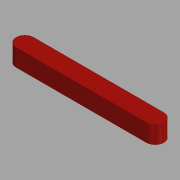
# Autodesk Inventor part: LED red
Saved by Autodesk Inventor 2014 SP2 (Build 180246200, 246)
## iProperties
Created: 2016-01-21
Part Number: LED red
Material: ABS plast
Document SubType Name: Modeling
Designer: Mervart
Mass: 0.0702602 g
Surface Area: 1.3885 cm^2
Volume: 0.0662832 cm^3
Density: 1.06 g/cm^3
Appearance: Oranžovo-červená
LastSaveDate: 21.09.2010
Hmotnost: 0
Author: Mervart
Autodesk Inventor part; units mm, degrees
ref_plane "YZ Plane" through (0, 0, 0) normal (1, 0, 0) x (0, 1, 0)
ref_plane "XZ Plane" through (0, 0, 0) normal (0, 1, 0) x (-1, 0, 0)
ref_plane "XY Plane" through (0, 0, 0) normal (0, 0, 1) x (1, 0, 0)
sketch "Náčrt4" plane through (0, 0, 0) normal (0, 0, 1) x (1, 0, 0)
  line L0 (-32.5599, -1.7649) -> (-17.5599, -1.7649) construction
  line L1 (-17.5599, -3.7649) -> (-32.5599, -3.7649) construction
  line L2 (-50.5599, -1.7649) -> (-35.5599, -1.7649) construction
  line L3 (-35.5599, -3.7649) -> (-50.5599, -3.7649) construction
  line L4 (-68.5599, -1.7649) -> (-53.5599, -1.7649) construction
  line L5 (-53.5599, -3.7649) -> (-68.5599, -3.7649) construction
  line L6 (-68.5599, 11.7351) -> (-9.4199, 11.7351) construction
  arc A0 (-68.5599, 11.7351) -> (-77.8599, 2.4351) centre (-68.5599, 2.4351) ccw construction
  line L7 (-77.8599, -87.5649) -> (-77.8599, 2.4351) construction
  arc A1 (-77.8599, -87.5649) -> (-68.5599, -96.8649) centre (-68.5599, -87.5649) ccw construction
  line L8 (-6.5599, -96.8649) -> (-68.5599, -96.8649) construction
  line L9 (-6.5599, -96.8649) -> (-6.5599, -2.5649) construction
  line L10 (-6.5599, -2.5649) -> (-9.4199, 11.7351) construction
  line L11 (-69.5599, -21.7649) -> (-69.5599, -7.7649) construction
  line L12 (-68.0599, -6.2649) -> (-54.0599, -6.2649) construction
  line L13 (-52.5599, -7.7649) -> (-52.5599, -21.7649) construction
  line L14 (-54.0599, -23.2649) -> (-68.0599, -23.2649) construction
  circle A2 centre (-43.0499, 7.9351) radius 0.3 construction
  circle A3 centre (-39.5499, 4.4351) radius 0.3 construction
  circle A4 centre (-43.0499, 0.9351) radius 0.3 construction
  circle A5 centre (-46.5499, 4.4351) radius 0.3 construction
  circle A6 centre (-43.0499, 4.4351) radius 0.3 construction
  circle A7 centre (-45.5248, 6.9099) radius 0.3 construction
  circle A8 centre (-45.5248, 1.9602) radius 0.3 construction
  circle A9 centre (-40.575, 1.9602) radius 0.3 construction
  circle A10 centre (-40.575, 6.9099) radius 0.3 construction
  line L15 (-32.5599, -1.7649) -> (-17.5599, -1.7649)
  line L16 (-17.5599, -3.7649) -> (-32.5599, -3.7649)
  line L17 (-38.3583, -87.0597) -> (-38.9319, -87.8789) projected
  arc A11 (-38.9319, -87.8789) -> (-47.1879, -87.8789) centre (-43.0599, -93.7743) ccw projected
  line L18 (-47.1879, -87.8789) -> (-47.7615, -87.0597) projected
  arc A12 (-38.3583, -87.0597) -> (-47.7615, -87.0597) centre (-43.0599, -93.7743) ccw projected
  circle A13 centre (-43.0599, -93.7743) radius 0.9 projected
  line L19 (-40.5363, -89.5777) -> (-41.1099, -90.3968) projected
  arc A14 (-41.1099, -90.3968) -> (-45.0099, -90.3968) centre (-43.0599, -93.7743) ccw projected
  line L20 (-45.0099, -90.3968) -> (-45.5835, -89.5777) projected
  arc A15 (-40.5363, -89.5777) -> (-45.5835, -89.5777) centre (-43.0599, -93.7743) ccw projected
  arc A16 (-36.4655, -84.3565) -> (-49.6543, -84.3565) centre (-43.0599, -93.7743) ccw projected
  line L21 (-36.4655, -84.3565) -> (-37.0391, -85.1757) projected
  arc A17 (-37.0391, -85.1757) -> (-49.0807, -85.1757) centre (-43.0599, -93.7743) ccw projected
  line L22 (-49.0807, -85.1757) -> (-49.6543, -84.3565) projected
  line L23 (-33.5599, -75.7649) -> (-33.5599, -61.7649) projected
  arc A18 (-32.0599, -60.2649) -> (-33.5599, -61.7649) centre (-32.0599, -61.7649) ccw projected
  line L24 (-32.0599, -60.2649) -> (-18.0599, -60.2649) projected
  arc A19 (-16.5599, -61.7649) -> (-18.0599, -60.2649) centre (-18.0599, -61.7649) ccw projected
  line L25 (-16.5599, -61.7649) -> (-16.5599, -75.7649) projected
  arc A20 (-18.0599, -77.2649) -> (-16.5599, -75.7649) centre (-18.0599, -75.7649) ccw projected
  line L26 (-18.0599, -77.2649) -> (-32.0599, -77.2649) projected
  arc A21 (-33.5599, -75.7649) -> (-32.0599, -77.2649) centre (-32.0599, -75.7649) ccw projected
  line L27 (-51.5599, -75.7649) -> (-51.5599, -61.7649) projected
  arc A22 (-50.0599, -60.2649) -> (-51.5599, -61.7649) centre (-50.0599, -61.7649) ccw projected
  line L28 (-50.0599, -60.2649) -> (-36.0599, -60.2649) projected
  arc A23 (-34.5599, -61.7649) -> (-36.0599, -60.2649) centre (-36.0599, -61.7649) ccw projected
  line L29 (-34.5599, -61.7649) -> (-34.5599, -75.7649) projected
  arc A24 (-36.0599, -77.2649) -> (-34.5599, -75.7649) centre (-36.0599, -75.7649) ccw projected
  line L30 (-36.0599, -77.2649) -> (-50.0599, -77.2649) projected
  arc A25 (-51.5599, -75.7649) -> (-50.0599, -77.2649) centre (-50.0599, -75.7649) ccw projected
  line L31 (-69.5599, -75.7649) -> (-69.5599, -61.7649) projected
  arc A26 (-68.0599, -60.2649) -> (-69.5599, -61.7649) centre (-68.0599, -61.7649) ccw projected
  line L32 (-68.0599, -60.2649) -> (-54.0599, -60.2649) projected
  arc A27 (-52.5599, -61.7649) -> (-54.0599, -60.2649) centre (-54.0599, -61.7649) ccw projected
  line L33 (-52.5599, -61.7649) -> (-52.5599, -75.7649) projected
  arc A28 (-54.0599, -77.2649) -> (-52.5599, -75.7649) centre (-54.0599, -75.7649) ccw projected
  line L34 (-54.0599, -77.2649) -> (-68.0599, -77.2649) projected
  arc A29 (-69.5599, -75.7649) -> (-68.0599, -77.2649) centre (-68.0599, -75.7649) ccw projected
  line L35 (-33.5599, -57.7649) -> (-33.5599, -43.7649) projected
  arc A30 (-32.0599, -42.2649) -> (-33.5599, -43.7649) centre (-32.0599, -43.7649) ccw projected
  line L36 (-32.0599, -42.2649) -> (-18.0599, -42.2649) projected
  arc A31 (-16.5599, -43.7649) -> (-18.0599, -42.2649) centre (-18.0599, -43.7649) ccw projected
  line L37 (-16.5599, -43.7649) -> (-16.5599, -57.7649) projected
  arc A32 (-18.0599, -59.2649) -> (-16.5599, -57.7649) centre (-18.0599, -57.7649) ccw projected
  line L38 (-18.0599, -59.2649) -> (-32.0599, -59.2649) projected
  arc A33 (-33.5599, -57.7649) -> (-32.0599, -59.2649) centre (-32.0599, -57.7649) ccw projected
  line L39 (-51.5599, -57.7649) -> (-51.5599, -43.7649) projected
  arc A34 (-50.0599, -42.2649) -> (-51.5599, -43.7649) centre (-50.0599, -43.7649) ccw projected
  line L40 (-50.0599, -42.2649) -> (-36.0599, -42.2649) projected
  arc A35 (-34.5599, -43.7649) -> (-36.0599, -42.2649) centre (-36.0599, -43.7649) ccw projected
  line L41 (-34.5599, -43.7649) -> (-34.5599, -57.7649) projected
  arc A36 (-36.0599, -59.2649) -> (-34.5599, -57.7649) centre (-36.0599, -57.7649) ccw projected
  line L42 (-36.0599, -59.2649) -> (-50.0599, -59.2649) projected
  arc A37 (-51.5599, -57.7649) -> (-50.0599, -59.2649) centre (-50.0599, -57.7649) ccw projected
  line L43 (-69.5599, -57.7649) -> (-69.5599, -43.7649) projected
  arc A38 (-68.0599, -42.2649) -> (-69.5599, -43.7649) centre (-68.0599, -43.7649) ccw projected
  line L44 (-68.0599, -42.2649) -> (-54.0599, -42.2649) projected
  arc A39 (-52.5599, -43.7649) -> (-54.0599, -42.2649) centre (-54.0599, -43.7649) ccw projected
  line L45 (-52.5599, -43.7649) -> (-52.5599, -57.7649) projected
  arc A40 (-54.0599, -59.2649) -> (-52.5599, -57.7649) centre (-54.0599, -57.7649) ccw projected
  line L46 (-54.0599, -59.2649) -> (-68.0599, -59.2649) projected
  arc A41 (-69.5599, -57.7649) -> (-68.0599, -59.2649) centre (-68.0599, -57.7649) ccw projected
  line L47 (-33.5599, -39.7649) -> (-33.5599, -25.7649) projected
  arc A42 (-32.0599, -24.2649) -> (-33.5599, -25.7649) centre (-32.0599, -25.7649) ccw projected
  line L48 (-32.0599, -24.2649) -> (-18.0599, -24.2649) projected
  arc A43 (-16.5599, -25.7649) -> (-18.0599, -24.2649) centre (-18.0599, -25.7649) ccw projected
  line L49 (-16.5599, -25.7649) -> (-16.5599, -39.7649) projected
  arc A44 (-18.0599, -41.2649) -> (-16.5599, -39.7649) centre (-18.0599, -39.7649) ccw projected
  line L50 (-18.0599, -41.2649) -> (-32.0599, -41.2649) projected
  arc A45 (-33.5599, -39.7649) -> (-32.0599, -41.2649) centre (-32.0599, -39.7649) ccw projected
  line L51 (-51.5599, -39.7649) -> (-51.5599, -25.7649) projected
  arc A46 (-50.0599, -24.2649) -> (-51.5599, -25.7649) centre (-50.0599, -25.7649) ccw projected
  line L52 (-50.0599, -24.2649) -> (-36.0599, -24.2649) projected
  arc A47 (-34.5599, -25.7649) -> (-36.0599, -24.2649) centre (-36.0599, -25.7649) ccw projected
  line L53 (-34.5599, -25.7649) -> (-34.5599, -39.7649) projected
  arc A48 (-36.0599, -41.2649) -> (-34.5599, -39.7649) centre (-36.0599, -39.7649) ccw projected
  line L54 (-36.0599, -41.2649) -> (-50.0599, -41.2649) projected
  arc A49 (-51.5599, -39.7649) -> (-50.0599, -41.2649) centre (-50.0599, -39.7649) ccw projected
  line L55 (-69.5599, -39.7649) -> (-69.5599, -25.7649) projected
  arc A50 (-68.0599, -24.2649) -> (-69.5599, -25.7649) centre (-68.0599, -25.7649) ccw projected
  line L56 (-68.0599, -24.2649) -> (-54.0599, -24.2649) projected
  arc A51 (-52.5599, -25.7649) -> (-54.0599, -24.2649) centre (-54.0599, -25.7649) ccw projected
  line L57 (-52.5599, -25.7649) -> (-52.5599, -39.7649) projected
  arc A52 (-54.0599, -41.2649) -> (-52.5599, -39.7649) centre (-54.0599, -39.7649) ccw projected
  line L58 (-54.0599, -41.2649) -> (-68.0599, -41.2649) projected
  arc A53 (-69.5599, -39.7649) -> (-68.0599, -41.2649) centre (-68.0599, -39.7649) ccw projected
  line L59 (-33.5599, -21.7649) -> (-33.5599, -7.7649) projected
  arc A54 (-32.0599, -6.2649) -> (-33.5599, -7.7649) centre (-32.0599, -7.7649) ccw projected
  line L60 (-32.0599, -6.2649) -> (-18.0599, -6.2649) projected
  arc A55 (-16.5599, -7.7649) -> (-18.0599, -6.2649) centre (-18.0599, -7.7649) ccw projected
  line L61 (-16.5599, -7.7649) -> (-16.5599, -21.7649) projected
  arc A56 (-18.0599, -23.2649) -> (-16.5599, -21.7649) centre (-18.0599, -21.7649) ccw projected
  line L62 (-18.0599, -23.2649) -> (-32.0599, -23.2649) projected
  arc A57 (-33.5599, -21.7649) -> (-32.0599, -23.2649) centre (-32.0599, -21.7649) ccw projected
  line L63 (-51.5599, -21.7649) -> (-51.5599, -7.7649) projected
  arc A58 (-50.0599, -6.2649) -> (-51.5599, -7.7649) centre (-50.0599, -7.7649) ccw projected
  line L64 (-50.0599, -6.2649) -> (-36.0599, -6.2649) projected
  arc A59 (-34.5599, -7.7649) -> (-36.0599, -6.2649) centre (-36.0599, -7.7649) ccw projected
  line L65 (-34.5599, -7.7649) -> (-34.5599, -21.7649) projected
  arc A60 (-36.0599, -23.2649) -> (-34.5599, -21.7649) centre (-36.0599, -21.7649) ccw projected
  line L66 (-36.0599, -23.2649) -> (-50.0599, -23.2649) projected
  arc A61 (-51.5599, -21.7649) -> (-50.0599, -23.2649) centre (-50.0599, -21.7649) ccw projected
  arc A62 (-32.5599, -1.7649) -> (-32.5599, -3.7649) centre (-32.5599, -2.7649) ccw projected
  arc A63 (-17.5599, -3.7649) -> (-17.5599, -1.7649) centre (-17.5599, -2.7649) ccw projected
  arc A64 (-50.5599, -1.7649) -> (-50.5599, -3.7649) centre (-50.5599, -2.7649) ccw projected
  arc A65 (-35.5599, -3.7649) -> (-35.5599, -1.7649) centre (-35.5599, -2.7649) ccw projected
  arc A66 (-68.5599, -1.7649) -> (-68.5599, -3.7649) centre (-68.5599, -2.7649) ccw projected
  arc A67 (-53.5599, -3.7649) -> (-53.5599, -1.7649) centre (-53.5599, -2.7649) ccw projected
  arc A68 (-68.0599, -6.2649) -> (-69.5599, -7.7649) centre (-68.0599, -7.7649) ccw projected
  arc A69 (-52.5599, -7.7649) -> (-54.0599, -6.2649) centre (-54.0599, -7.7649) ccw projected
  arc A70 (-54.0599, -23.2649) -> (-52.5599, -21.7649) centre (-54.0599, -21.7649) ccw projected
  arc A71 (-69.5599, -21.7649) -> (-68.0599, -23.2649) centre (-68.0599, -21.7649) ccw projected
  point P0 (0, 0)
  point P1 (-16.5599, -2.7649)
  constraints: 5 point on circle, 4 end point, 1 horizontal, 1 parallel
extrude "Vysunutí1" add sketch "Náčrt4" against normal blind 2 contours L15 A63 L16 A62
